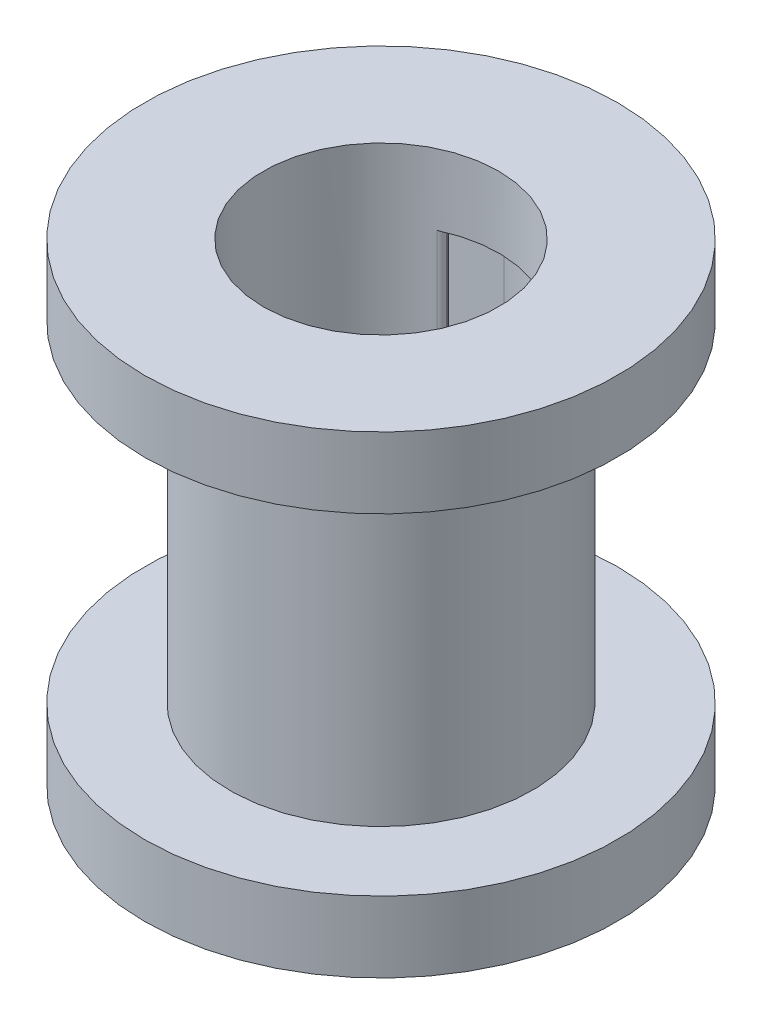
# Autodesk Inventor part: Spring Spool
Saved by Autodesk Inventor 2023.2 (Build 272271000, 271)
## iProperties
Created: 2024-03-24
Part Number: Spring Spool
Material: Nylon 6/6
Document SubType Name: Modeling
Designer: Nathan Cai
Density: 1.13 g/cm^3
Appearance: Nylon 6
Author: Nathan Cai
Autodesk Inventor part; units mm, degrees
ref_plane "YZ Plane" through (0, 0, 0) normal (1, 0, 0) x (0, 1, 0)
ref_plane "XZ Plane" through (0, 0, 0) normal (0, 1, 0) x (-1, 0, 0)
ref_plane "XY Plane" through (0, 0, 0) normal (0, 0, 1) x (1, 0, 0)
sketch "Sketch1" plane through (0, 0, 0) normal (1, 0, 0) x (0, 1, 0)
  line L0 (0, 0) -> (15.875, 0)
  line L1 (15.875, 0) -> (15.875, 5.08)
  line L2 (15.875, 5.08) -> (0, 5.08)
  line L3 (0, 5.08) -> (0, 0)
  line L4 (15.875, 5.08) -> (13.49375, 5.08)
  line L5 (13.49375, 5.08) -> (13.49375, 7.9375)
  line L6 (13.49375, 7.9375) -> (15.875, 7.9375)
  line L7 (15.875, 7.9375) -> (15.875, 5.08)
  line L8 (0, 5.08) -> (2.38125, 5.08)
  line L9 (2.38125, 5.08) -> (2.38125, 7.9375)
  line L10 (2.38125, 7.9375) -> (0, 7.9375)
  line L11 (0, 7.9375) -> (0, 5.08)
  line L12 (15.875, 3.95) -> (0, 3.95)
  line L13 (0, 3.95) -> (0, 0)
  line L14 (0, 0) -> (15.875, 0)
  line L15 (15.875, 0) -> (15.875, 3.95)
  point P0 (0, 3.95)
  dimension "d0" = 15.875
  dimension "d1" = 5.08
  dimension "d2" = 2.38125
  dimension "d3" = 2.38125
  dimension "d4" = 7.9375
  dimension "d5" = 3.95
  constraints: 32 end point, 8 parallel, 4 horizontal, 4 perpendicular, 2 point on line
  measures "d0" distance of L2.end L1.end
  measures "d1" distance of L1.end L0.end
  measures "d2" distance of L5.end L6.end
  measures "d3" distance of L10.end L9.end
  measures "d4" distance between parallel lines of L0 L6
  measures "d5" distance between parallel lines of L0 L12
sketch "Sketch1 outline for Revolution1" plane through (0, 0, 0) normal (1, 0, 0) x (0, 1, 0)
  line L0 (15.875, 5.08) -> (15.875, 7.9375)
  line L1 (15.875, 3.95) -> (15.875, 5.08)
  line L2 (0, 3.95) -> (15.875, 3.95)
  line L3 (0, 5.08) -> (0, 3.95)
  line L4 (0, 7.9375) -> (0, 5.08)
  line L5 (2.38125, 7.9375) -> (0, 7.9375)
  line L6 (2.38125, 5.08) -> (2.38125, 7.9375)
  line L7 (13.49375, 5.08) -> (2.38125, 5.08)
  line L8 (13.49375, 7.9375) -> (13.49375, 5.08)
  line L9 (15.875, 7.9375) -> (13.49375, 7.9375)
revolve "Revolution1" add sketch "Sketch1 outline for Revolution1" angle 360 about axis through (0, 0, 0) along (0, 1, 0)
sketch "Sketch2" plane through (0, 2.38125, 0) normal (0, 1, 0) x (1, 0, 0)
  circle A0 centre (0, 0) radius 3.95
  circle A1 centre (0, 0) radius 4.1278
  line L0 (3.95, 0) -> (4.1278, 0)
  line L1 (0, 3.95) -> (0, 4.1278)
  circle A2 centre (0, 0) radius 5.08
  line L2 (0, 4.1278) -> (-3.194354, 4.1278)
  line L3 (-3.194354, 4.1278) -> (-3.194354, 3.95)
  line L4 (-3.194354, 3.95) -> (0, 3.95)
  line L5 (0, 3.95) -> (0, 4.1278)
  point P0 (0, 0)
  dimension "d7" = 0.1778
  constraints: 12 end point, 4 point on circle, 3 point on line, 2 horizontal, 2 parallel, 2 perpendicular, 1 centre point, 2 other
  measures "d7" radial gap between concentric circles of A0 A1
sketch "Sketch2 outline for Extrusion1" plane through (0, 2.38125, 0) normal (0, 1, 0) x (1, 0, 0)
  line L0 (-3.194354, 3.95) -> (0, 3.95)
  line L1 (-3.194354, 4.1278) -> (-3.194354, 3.95)
  line L2 (0, 4.1278) -> (-3.194354, 4.1278)
  arc A0 (4.1278, 0) -> (0, 4.1278) centre (0, 0) ccw
  line L3 (3.95, 0) -> (4.1278, 0)
  arc A1 (0, 3.95) -> (3.95, 0) centre (0, 0) cw
extrude "Extrusion1" cut sketch "Sketch2 outline for Extrusion1" along normal up to surface (11.1125 mm away)
ref_plane "Work Plane1" through (3.95, 7.9375, 0) normal (0.7071068, 0, -0.7071068) x (0, -1, 0)
sketch "Sketch3" plane through (3.95, 7.9375, 0) normal (0.7071068, 0, -0.7071068) x (0, -1, 0)
  line L0 (7.9375, 2.793072) -> (-7.9375, 2.793072) construction
  line L1 (-7.9375, 6.743072) -> (-7.9375, -1.156928)
  circle A0 centre (0, 2.793072) radius 1.651
  dimension "d12" = 3.302
  constraints: 2 end point, 2 midpoint, 1 centre point
  measures "d12" diameter of A0
sketch "Sketch3 outline for Extrusion2" plane through (3.95, 7.9375, 0) normal (0.7071068, 0, -0.7071068) x (0, -1, 0)
  circle A0 centre (0, 2.793072) radius 1.651
extrude "Extrusion2" add sketch "Sketch3 outline for Extrusion2" along normal blind 1.5875
sketch "Sketch4" plane through (0, 0, 0) normal (0, -1, 0) x (1, 0, 0)
  circle A0 centre (0, 0) radius 3.95 projected
  point P0 (0, 0)
sketch "Sketch4 outline for Extrusion3" plane through (0, 0, 0) normal (0, -1, 0) x (1, 0, 0)
  circle A0 centre (0, 0) radius 3.95
extrude "Extrusion3" cut sketch "Sketch4 outline for Extrusion3" against normal through all
fillet "Fillet1" radius 0.198437 2 edges at (0, 7.9375, -3.95) (-2.961, 7.9375, -4.1278)
fillet "Fillet2" radius 3.175 1 edges at (-3.1944, 7.9375, -3.95)
equation "\"d3\" = d2"
body "Solid1"
